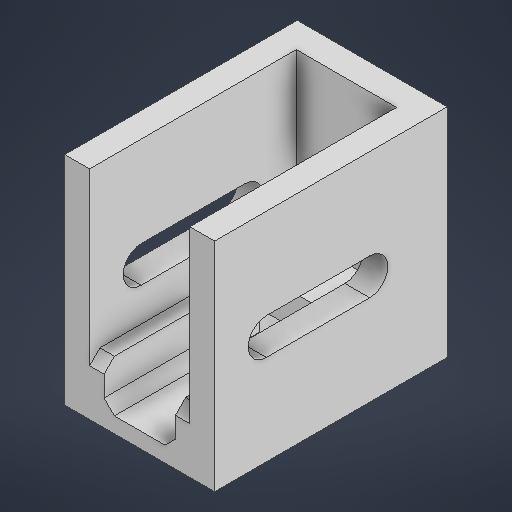
# Autodesk Inventor part: tensionerholder
Saved by Autodesk Inventor 2025.1 (Build 291241000, 241)
## iProperties
Created: 2025-02-02
Part Number: tensionerholder
Material: Generic
Document SubType Name: Modeling
Designer: jerem
Density: 1 g/cm^3
Appearance: Default
Author: jerem
## iProperties of the stored document tensionerholder_3DPrint.ipt
Created: 2025-02-02
Part Number: tensionerholder_3DPrint
Material: Generic
Document SubType Name: Modeling
Designer: jerem
Density: 1 g/cm^3
Appearance: Default
Author: jerem
Autodesk Inventor part; units mm, degrees
ref_plane "YZ Plane" through (0, 0, 0) normal (1, 0, 0) x (0, 1, 0)
ref_plane "XZ Plane" through (0, 0, 0) normal (0, 1, 0) x (-1, 0, 0)
ref_plane "XY Plane" through (0, 0, 0) normal (0, 0, 1) x (1, 0, 0)
sketch "Sketch1" plane through (0, 0, 0) normal (0, 1, 0) x (-1, 0, 0)
  line L0 (9.7, 0) -> (9.7, -40)
  line L1 (9.7, -40) -> (-9.7, -40)
  line L2 (-9.7, -40) -> (-9.7, 0)
  line L3 (-9.7, 0) -> (0, 0)
  line L4 (0, 0) -> (9.7, 0)
  line L5 (-9.7, 0) -> (-14.5, 0)
  line L6 (-14.5, 0) -> (-14.5, -45)
  line L7 (-14.5, -45) -> (14.5, -45)
  line L8 (14.5, -45) -> (14.5, 0)
  line L9 (14.5, 0) -> (9.7, 0)
  line L10 (6.9, 0) -> (6.9, -30)
  line L11 (6.9, -30) -> (-6.9, -30)
  line L12 (-6.9, -30) -> (-6.9, 0)
  line L13 (-6.9, -30) -> (-9.7, -30) construction
  line L14 (6.9, -30) -> (9.7, -30) construction
  dimension "d0" = 40
  dimension "d1" = 19.4
  dimension "d2" = 5
  dimension "d16" = 2.8
  dimension "d17" = 10
  dimension "d26" = 29
  constraints: 30 end point, 9 perpendicular, 6 point on line, 4 collinear, 2 horizontal, 2 vertical
  measures "d0" distance of L0.start L0.end
  measures "d1" distance of L0.end L1.end
  measures "d2" distance between parallel lines of L7 L1
  measures "d16" distance of L10.end L14.end
  measures "d17" distance between parallel lines of L1 L11
  measures "d26" distance between parallel lines of L6 L8
extrude "Extrusion1" add sketch "Sketch1" along normal blind 42 contours L9 L8 L7 L6 L5 L2 L1 L0
sketch "Sketch2" plane through (14.5, 0, 0) normal (1, 0, 0) x (0, 0, -1)
  line L0 (0, 0) -> (45, 0) projected
  line L1 (45, 0) -> (45, 42) projected
  line L2 (0, 42) -> (45, 42) projected
  line L3 (0, 0) -> (0, 42) projected
  line L4 (0, 21) -> (10, 21) construction
  circle A0 centre (10, 21) radius 3.5
  line L5 (10, 21) -> (30, 21) construction
  circle A1 centre (30, 21) radius 3.5
  line L6 (10, 24.5) -> (30, 24.5)
  line L7 (30, 17.5) -> (10, 17.5)
  point P0 (0, 0)
  dimension "d6" = 7
  dimension "d7" = 20
  dimension "d8" = 10
  constraints: 8 end point, 4 point on circle, 4 tangent, 2 centre point, 2 coincident, 2 horizontal, 1 equal radius, 1 midpoint
  measures "d6" diameter of A0
  measures "d7" distance of L5.end L4.end
  measures "d8" distance from line of L3 L4.end
extrude "Extrusion2" cut sketch "Sketch2" against normal through all contours A0 | A0 L6 A1 L7 | A1
sketch "Sketch3" plane through (14.5, 0, -45) normal (0, 0, -1) x (-1, 0, 0)
  line L0 (0, 0) -> (29, 0) projected
  line L1 (29, 0) -> (29, 42) projected
  line L2 (0, 42) -> (29, 42) projected
  line L3 (0, 0) -> (0, 42) projected
  line L4 (29, 0) -> (29, 42) construction
  line L5 (29, 21) -> (14.5, 21) construction
  line L6 (14.5, 21) -> (14.5, 0) construction
  circle A0 centre (14.5, 21) radius 1.7
  dimension "d11" = 3.4
  constraints: 4 end point, 2 perpendicular, 1 centre point, 1 coincident, 1 midpoint
  measures "d11" diameter of A0
extrude "Extrusion3" cut sketch "Sketch3" against normal blind 10 contours A0
extrude "Extrusion4" add sketch "Sketch1" along normal blind 11 contours L0 L1 L2 L3 L12 L11 L10 L4
extrude "Extrusion5" add sketch "Sketch1" along normal blind 3 contours L10 L11 L12 L3 L4
chamfer "Chamfer1" distance 2 angle 45 3 edges at (-6.9, 3, -15) (0, 3, -30) (6.9, 3, -15)
chamfer "Chamfer2" distance 2 angle 45 2 edges at (-8.3, 11, 0) (8.3, 11, 0)
body "Solid1"
